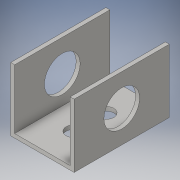
# Autodesk Inventor part: Scaling Arms Mounting Bracket
Saved by Autodesk Inventor 2016 (Build 200138000, 138)
## iProperties
Created: 2016-01-30
Part Number: Scaling Arms Mounting Bracket
Material: Generic
Document SubType Name: Modeling
Designer: gus
Density: 1 g/cm^3
Appearance: Default
Author: gus
Autodesk Inventor part; units mm, degrees
ref_plane "YZ Plane" through (0, 0, 0) normal (1, 0, 0) x (0, 1, 0)
ref_plane "XZ Plane" through (0, 0, 0) normal (0, 1, 0) x (-1, 0, 0)
ref_plane "XY Plane" through (0, 0, 0) normal (0, 0, 1) x (1, 0, 0)
sketch "Sketch1" plane through (0, 0, 0) normal (0, 1, 0) x (-1, 0, 0)
  line L0 (0, 0) -> (50.8, 0)
  line L1 (50.8, 0) -> (50.8, -76.2)
  line L2 (50.8, -76.2) -> (0, -76.2)
  line L3 (0, -76.2) -> (0, 0)
  circle A0 centre (25.4, -50.8) radius 6.35
  circle A1 centre (25.4, -25.4) radius 6.35
  dimension "d0" = 50.8
  dimension "d1" = 76.2
  dimension "d13" = 25.4
  dimension "d14" = 25.4
  dimension "d15" = 25.4
  dimension "d16" = 25.4
  dimension "d17" = 12.7
  dimension "d18" = 12.7
  constraints: 8 end point, 2 centre point, 2 parallel, 1 horizontal, 1 perpendicular
  measures "d0" distance of L1.end L2.end
  measures "d1" distance of L2.end L0.start
  measures "d13" distance from line of L2 A0.centre
  measures "d14" distance from line of L1 A0.centre
  measures "d15" distance from line of L0 A1.centre
  measures "d16" distance from line of L1 A1.centre
  measures "d17" diameter of A0
  measures "d18" diameter of A1
extrude "Extrusion3" add sketch "Sketch1" along normal blind 3.175
sketch "Sketch5" plane through (0, 3.175, 0) normal (0, 1, 0) x (1, 0, 0)
  line L0 (0, 76.2) -> (-50.8, 76.2) projected
  line L1 (-50.8, 76.2) -> (-47.625, 76.2)
  line L2 (-47.625, 76.2) -> (-47.625, 0)
  line L3 (-47.625, 0) -> (-50.8, 0)
  line L4 (-50.8, 0) -> (-50.8, 76.2)
  line L5 (0, 76.2) -> (-3.175, 76.2)
  line L6 (-3.175, 76.2) -> (-3.175, 0)
  line L7 (-3.175, 0) -> (0, 0)
  line L8 (0, 0) -> (0, 76.2)
  point P0 (0, 0)
  dimension "d21" = 3.175
  dimension "d22" = 3.175
  dimension "d23" = 76.2
  dimension "d24" = 76.2
  constraints: 16 end point, 4 parallel, 2 horizontal, 2 perpendicular
  measures "d21" distance of L2.end L3.end
  measures "d22" distance of L7.end L6.end
  measures "d23" distance of L5.end L6.end
  measures "d24" distance of L1.end L2.end
extrude "Extrusion4" add sketch "Sketch5" along normal blind 47.625
sketch "Sketch6" plane through (-50.8, 0, -76.2) normal (-1, 0, 0) x (0, 0, 1)
  circle A0 centre (38.1, 25.4) radius 14.2748
  line L0 (76.2, 0) -> (76.2, 50.8) projected
  line L1 (76.2, 0) -> (0, 0) projected
  dimension "d27" = 28.5496
  dimension "d28" = 38.1
  dimension "d29" = 25.4
  constraints: 1 centre point
  measures "d27" diameter of A0
  measures "d28" distance from line of L0 A0.centre
  measures "d29" distance from line of L1 A0.centre
extrude "Extrusion6" cut sketch "Sketch6" against normal blind 50.8
equation "\"d24\" = d23"
body "Solid2"
